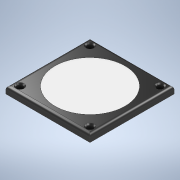
# Autodesk Inventor part: Filter
Saved by Autodesk Inventor 2020 (Build 240168000, 168)
## iProperties
Created: 2019-12-12
Part Number: Filter
Material: Generic
Document SubType Name: Modeling
Designer: nicoc
Density: 1 g/cm^3
Appearance: Glossy - Black
Author: nicoc
Autodesk Inventor part; units mm, degrees
ref_plane "YZ Plane" through (0, 0, 0) normal (1, 0, 0) x (0, 1, 0)
ref_plane "XZ Plane" through (0, 0, 0) normal (0, 1, 0) x (-1, 0, 0)
ref_plane "XY Plane" through (0, 0, 0) normal (0, 0, 1) x (1, 0, 0)
sketch "Sketch1" plane through (0, 0, 0) normal (0, 1, 0) x (-1, 0, 0)
  line L0 (0, 0) -> (60, 0)
  line L1 (60, 0) -> (60, -60)
  line L2 (60, -60) -> (0, -60)
  line L3 (0, -60) -> (0, 0)
  dimension "d0" = 60
  dimension "d1" = 60
  constraints: 8 end point, 2 parallel, 1 horizontal, 1 perpendicular
  measures "d0" distance between parallel lines of L2 L0
  measures "d1" distance between parallel lines of L1 L3
extrude "Extrusion1" add sketch "Sketch1" along normal blind 5
sketch "Sketch2" plane through (0, 5, 0) normal (0, 1, 0) x (1, 0, 0)
  line L0 (-60, 0) -> (0, 0) projected
  line L1 (0, 0) -> (0, 60) projected
  line L2 (0, 60) -> (-60, 60) projected
  line L3 (-60, 60) -> (-60, 0) projected
  point P0 (-5, 5)
  point P1 (-5, 55)
  point P2 (-55, 55)
  point P3 (-55, 5)
  dimension "d4" = 5
  dimension "d6" = 5
  dimension "d7" = 5
  dimension "d8" = 5
  dimension "d9" = 5
  dimension "d10" = 5
  dimension "d11" = 5
  dimension "d12" = 5
  measures "d4" distance from line of point (-5, 5) L0
  measures "d6" distance from line of point (-5, 5) L1
  measures "d7" distance from line of L1 point (-5, 55)
  measures "d8" distance from line of L2 point (-55, 55)
  measures "d9" distance from line of L3 point (-55, 55)
  measures "d10" distance from line of point (-55, 5) L0
  measures "d11" distance from line of L3 point (-55, 5)
  measures "d12" distance from line of point (-5, 55) L2
hole "Hole1" at (-5, 5, -5) at (-5, 5, -55) at (-55, 5, -55) at (-55, 5, -5) direction (0, -1, 0) diameter 4.3 end through all countersink diameter 6 countersink angle 90
fillet "Fillet1" radius 2 4 edges at (-30, 5, 0) (-60, 5, -30) (-30, 5, -60) (0, 5, -30)
sketch "Sketch3" plane through (0, 5, 0) normal (0, 1, 0) x (1, 0, 0)
  circle A0 centre (-30, 30) radius 25
  line L0 (-60, 0) -> (0, 0) projected
  line L1 (-60, 60) -> (-60, 0) projected
  dimension "d21" = 30
  dimension "d22" = 30
  dimension "d23" = 50
  constraints: 1 centre point
  measures "d21" distance from line of A0.centre L0
  measures "d22" distance from line of A0.centre L1
  measures "d23" diameter of A0
extrude "Extrusion2" cut sketch "Sketch3" against normal blind 0.1
body "Solid1"
